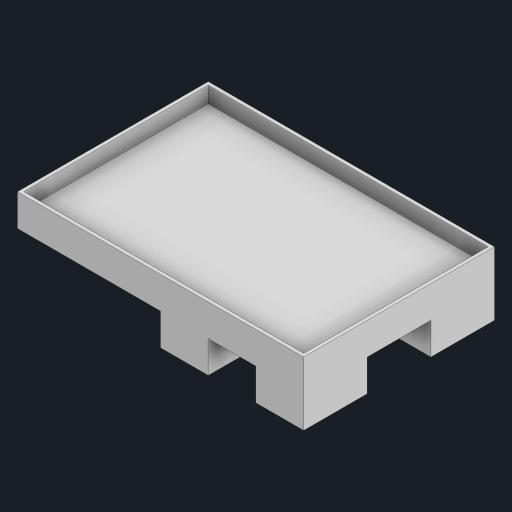
# Autodesk Inventor part: table_bed
Saved by Autodesk Inventor 2024 (Build 280153000, 153)
## iProperties
Created: 2024-06-21
Part Number: table_bed
Material: Generic
Document SubType Name: Modeling
Designer: mihir
Density: 1 g/cm^3
Appearance: Default
Author: mihir
Autodesk Inventor part; units mm, degrees
ref_plane "YZ Plane" through (0, 0, 0) normal (1, 0, 0) x (0, 1, 0)
ref_plane "XZ Plane" through (0, 0, 0) normal (0, 1, 0) x (-1, 0, 0)
ref_plane "XY Plane" through (0, 0, 0) normal (0, 0, 1) x (1, 0, 0)
sketch "Sketch1" plane through (0, 0, 0) normal (0, 1, 0) x (-1, 0, 0)
  line L0 (0, 0) -> (180, 0)
  line L1 (180, 0) -> (180, -120)
  line L2 (180, -120) -> (0, -120)
  line L3 (0, -120) -> (0, 0)
  dimension "d0" = 120
  dimension "d1" = 180
  constraints: 8 end point, 2 parallel, 1 horizontal, 1 perpendicular
  measures "d0" distance of L2.end L0.start
  measures "d1" distance of L0.start L0.end
extrude "Extrusion1" add sketch "Sketch1" along normal blind 20
sketch "Sketch2" plane through (0, 20, 0) normal (0, 1, 0) x (1, 0, 0)
  line L0 (-178, 2) -> (-2, 2)
  line L1 (-2, 2) -> (-2, 118)
  line L2 (-2, 118) -> (-178, 118)
  line L3 (-178, 118) -> (-178, 2)
  line L4 (-180, 120) -> (-180, 0) projected
  line L5 (-180, 0) -> (0, 0) projected
  dimension "d4" = 2
  dimension "d5" = 2
  dimension "d6" = 176
  dimension "d7" = 116
  constraints: 8 end point, 2 parallel, 1 horizontal, 1 perpendicular
  measures "d4" distance between parallel lines of L4 L3
  measures "d5" distance between parallel lines of L5 L0
  measures "d6" distance of L0.start L0.end
  measures "d7" distance of L2.end L0.start
extrude "Extrusion2" cut sketch "Sketch2" against normal blind 10
sketch "Sketch3" plane through (0, 0, 0) normal (0, -1, 0) x (1, 0, 0)
  line L0 (0, 0) -> (-30, 0)
  line L1 (-30, 0) -> (-30, -40)
  line L2 (-30, -40) -> (0, -40)
  line L3 (0, -40) -> (0, 0)
  dimension "d10" = 30
  dimension "d11" = 40
  constraints: 8 end point, 2 parallel, 1 horizontal, 1 perpendicular
  measures "d10" distance of L1.end L2.end
  measures "d11" distance of L0.end L1.end
extrude "Extrusion3" add sketch "Sketch3" along normal blind 20
sketch "Sketch4" plane through (0, -20, 0) normal (0, -1, 0) x (1, 0, 0)
  line L0 (-5, -5) -> (-25, -5)
  line L1 (-25, -5) -> (-25, -10)
  line L2 (-25, -10) -> (-5, -10)
  line L3 (-5, -10) -> (-5, -5)
  line L4 (0, -40) -> (0, 0) projected
  line L5 (-5, -5) -> (0, -5) construction
  line L6 (0, 0) -> (-30, 0) construction
  dimension "d14" = 5
  dimension "d15" = 20
  dimension "d16" = 5
  dimension "d17" = 5
  constraints: 10 end point, 2 parallel, 2 perpendicular, 1 horizontal, 1 point on line
  measures "d14" distance of L2.end L0.start
  measures "d15" distance of L0.start L0.end
  measures "d16" distance between parallel lines of L4 L3
  measures "d17" distance between parallel lines of L6 L0
revolve "Revolution1" cut sketch "Sketch4" angle 360 about axis through (-25, -20, -10) along (1, 0, 0)
sketch "Sketch5" plane through (0, -20, 0) normal (0, -1, 0) x (1, 0, 0)
  line L0 (-30, -40) -> (0, -40) projected
  line L1 (-10, -20) -> (-20, -20) construction
  line L2 (-15, -20) -> (-15, -40) construction
  point P0 (0, 0)
  dimension "d19" = 10
  dimension "d20" = 20
  constraints: 4 end point, 2 midpoint, 1 horizontal, 1 vertical
  measures "d19" distance of L1.end L1.start
  measures "d20" distance from line of L0 L1.start
hole "Hole1" at (-10, -20, -20) at (-20, -20, -20) direction (0, 1, 0) diameter 1 depth 20 tip angle 118
ref_plane "Work Plane1" through (-180, 20, -60) normal (0, 0, 1) x (1, 0, 0)
ref_plane "Work Plane2" through (-90, 0, -120) normal (1, 0, 0) x (0, 0, -1)
mirror "Mirror1" about plane through (-180, 20, -60) normal (0, 0, 1) of "Extrusion3", "Revolution1", "Hole1"
ref_plane "Work Plane3" through (-45, 0, -120) normal (1, 0, 0) x (0, 0, -1)
mirror "Mirror2" about plane through (-45, 0, -120) normal (1, 0, 0) of "Extrusion3", "Revolution1", "Hole1", "Mirror1"
equation "\"d0\" = table_bed_width"
equation "\"d1\" = table_bed_length"
equation "\"d2\" = table_bed_thickness"
equation "\"d4\" = table_bed_wall_thickness"
equation "\"d5\" = table_bed_wall_thickness"
equation "\"d6\" = table_bed_length - 2 * table_bed_wall_thickness"
equation "\"d7\" = table_bed_width - 2 * table_bed_wall_thickness"
equation "\"d8\" = table_bed_indent_depth"
equation "\"d10\" = table_bed_peg_width"
equation "\"d11\" = table_bed_peg_length"
equation "\"d12\" = table_bed_peg_height"
equation "\"d14\" = 0.5 * bearing_diameter"
equation "\"d15\" = bearing_length"
equation "\"d16\" = 0.5 * table_bed_peg_width - 0.5 * bearing_length"
equation "\"d17\" = 0.5 * table_bed_peg_width - 0.5 * bearing_length"
equation "\"d19\" = screw_x"
equation "\"d20\" = screw_y"
equation "\"d21\" = screw_diameter"
equation "\"table_bed_width\" = 120"
equation "\"table_bed_length\" = 180"
equation "\"table_bed_thickness\" = 20"
equation "\"table_bed_indent_depth\" = 10"
equation "\"table_bed_wall_thickness\" = 2"
equation "\"screw_diameter\" = 1"
equation "\"table_bed_peg_length\" = 40"
equation "\"table_bed_peg_width\" = 30"
equation "\"table_bed_peg_height\" = 20"
equation "\"bearing_length\" = 20"
equation "\"screw_x\" = 10"
equation "\"screw_y\" = 20"
equation "\"bearing_diameter\" = 10"
body "Solid1"
